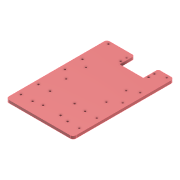
# Autodesk Inventor part: base plate
Saved by Autodesk Inventor 2022 (Build 260153000, 153)
## iProperties
Created: 2024-03-20
Part Number: base plate
Material: Generic
Document SubType Name: Modeling
Designer: david
Density: 1 g/cm^3
Appearance: Smooth - Red
Author: david
Autodesk Inventor part; units mm, degrees
ref_plane "YZ Plane" through (0, 0, 0) normal (1, 0, 0) x (0, 1, 0)
ref_plane "XZ Plane" through (0, 0, 0) normal (0, 1, 0) x (-1, 0, 0)
ref_plane "XY Plane" through (0, 0, 0) normal (0, 0, 1) x (1, 0, 0)
sketch "Sketch1" plane through (0, 0, 0) normal (0, 1, 0) x (-1, 0, 0)
  line L0 (57.5, -173) -> (57.5, -173) construction
  line L1 (-57.5, -173) -> (-57.5, 0) construction
  line L2 (-57.5, 0) -> (57.5, 0)
  line L3 (57.5, 0) -> (57.5, -173) construction
  line L4 (80.5, 0) -> (-80.5, 0) construction
  line L5 (0, -207.6) -> (0, 34.6) construction
  line L6 (57.5, -173) -> (-57.5, -173)
  line L7 (-57.5, -173) -> (-57.5, -173) construction
  line L8 (-57.5, 0) -> (57.5, 0)
  line L9 (57.5, 0) -> (57.5, -40)
  line L10 (-57.5, -40) -> (-57.5, 0)
  line L11 (57.5, -40) -> (57.5, -173)
  line L12 (-57.5, -173) -> (-57.5, -40)
  point P0 (0, 0)
  dimension "width" = 115
  dimension "Length" = 173
  dimension "d2" = 115
  constraints: 22 end point, 5 parallel, 4 horizontal, 4 perpendicular, 1 collinear, 1 point on line, 1 symmetric about line, 1 vertical alignment, 1 other
  measures "width" distance of L1.end L2.end
  measures "Length" distance of L1.start L1.end
  measures "d2" distance of L6.end L0.end
extrude "Base" add sketch "Sketch1" against normal blind 5
sketch "Sketch2" plane through (0, 0, 0) normal (0, 1, 0) x (1, 0, 0)
  line L0 (30, 48) -> (50, 48) construction
  line L1 (50, 48) -> (50, 18) construction
  line L2 (50, 18) -> (30, 18) construction
  line L3 (30, 18) -> (30, 48) construction
  line L4 (0, 207.6) -> (0, -34.6) construction
  line L5 (-30, 48) -> (-50, 48) construction
  line L6 (-50, 48) -> (-50, 18) construction
  line L7 (-50, 18) -> (-30, 18) construction
  line L8 (-30, 18) -> (-30, 48) construction
  line L9 (-57.5, 0) -> (57.5, 0) projected
  line L10 (-35, 53) -> (-25, 53) construction
  line L11 (-25, 53) -> (-25, 13) construction
  line L12 (-25, 13) -> (-35, 13) construction
  line L13 (-35, 13) -> (-35, 53) construction
  line L14 (-30, 43) -> (-30, 23) construction
  line L15 (30, 18) -> (30, 48) construction
  line L16 (35, 53) -> (25, 53) construction
  line L17 (25, 53) -> (25, 13) construction
  line L18 (25, 13) -> (35, 13) construction
  line L19 (35, 13) -> (35, 53) construction
  line L20 (30, 43) -> (30, 23) construction
  point P0 (0, 0)
  point P1 (-30, 53)
  point P2 (-30, 33)
  point P3 (-25, 33)
  point P4 (-30, 33)
  point P5 (30, 53)
  point P6 (30, 33)
  point P7 (25, 33)
  point P8 (30, 33)
  dimension "d5" = 20
  dimension "d6" = 30
  dimension "d8" = 18
  dimension "d16" = 10
  dimension "d18" = 20
  dimension "d19" = 10
  dimension "d20" = 50
  constraints: 38 end point, 18 symmetric about line, 8 coincident, 4 midpoint, 4 parallel, 4 point on line, 2 horizontal, 2 perpendicular, 1 horizontal alignment, 1 vertical alignment
  measures "d5" distance of L1.end L2.end
  measures "d6" distance of L0.end L1.end
  measures "d8" distance between parallel lines of L9 L2
  measures "d16" distance of L10.start L10.end
  measures "d18" distance of L14.end L14.start
  measures "d19" vertical distance of L10.end L14.start
  measures "d20" distance between parallel lines of L17 L11
hole "Bearing Holder Mounting Holes" at (30, 0, -48) at (50, 0, -48) at (50, 0, -18) at (-50, 0, -18) at (-30, 0, -48) at (-50, 0, -48) at (-30, 0, -18) at (30, 0, -18) direction (0, -1, 0) diameter 3.4 end through all
fillet "Fillet1" radius 5 4 edges at (57.5, -2.5, 0) (57.5, -2.5, -173) (-57.5, -2.5, -173) (-57.5, -2.5, 0)
sketch "Sketch5" plane through (0, 0, 0) normal (0, 1, 0) x (1, 0, 0)
  line L0 (-34.5, 80) -> (34.5, 80) construction
  line L1 (34.5, 80) -> (34.5, 114) construction
  line L2 (34.5, 114) -> (-34.5, 114) construction
  line L3 (-34.5, 114) -> (-34.5, 80) construction
  line L4 (-57.5, 0) -> (52.5, 0) projected
  point P0 (0, 0)
  point P1 (-52.2987, 0)
  point P2 (0, 80)
  dimension "d41" = 34
  dimension "d42" = 69
  dimension "d43" = 80
  constraints: 8 end point, 2 parallel, 1 horizontal, 1 midpoint, 1 perpendicular, 1 vertical alignment
  measures "d41" distance of L2.end L0.start
  measures "d42" distance of L1.end L2.end
  measures "d43" distance between parallel lines of L4 L0
hole "12v Motor Mount Mounting Holes" at (-34.5, 0, -114) at (-34.5, 0, -80) at (34.5, 0, -80) at (34.5, 0, -114) direction (0, -1, 0) diameter 3.2 end through all
sketch "Sketch8" plane through (0, 0, 0) normal (0, 1, 0) x (1, 0, 0)
  line L0 (-10, 148) -> (30, 148)
  line L1 (30, 148) -> (30, 168)
  line L2 (30, 168) -> (-10, 168)
  line L3 (-10, 168) -> (-10, 148)
  line L4 (52.5, 173) -> (-52.5, 173) projected
  line L5 (-57.5, 0) -> (52.5, 0) projected
  line L6 (-52.5, 173) -> (52.5, 173) projected
  line L7 (-10, 168) -> (30, 168)
  line L8 (30, 168) -> (30, 173)
  line L9 (30, 173) -> (-10, 173)
  line L10 (-10, 173) -> (-10, 168)
  point P0 (0, 0)
  point P1 (0, 173)
  point P2 (30, 170.5)
  dimension "d64" = 20
  dimension "d65" = 40
  dimension "d67" = 10
  dimension "d147" = 5
  constraints: 16 end point, 4 parallel, 2 horizontal, 2 midpoint, 2 perpendicular, 1 point on line, 1 vertical alignment
  measures "d64" distance of L2.end L0.start
  measures "d65" distance of L1.end L2.end
  measures "d67" distance from line of point (0, 173) L3
  measures "d147" distance between parallel lines of L4 L2
extrude "Servo Cutout 2" cut sketch "Sketch8" against normal through all
sketch "Sketch9" plane through (0, 0, 0) normal (0, 1, 0) x (1, 0, 0)
  line L0 (-13.925, 153) -> (33.925, 153) construction
  line L1 (33.925, 153) -> (33.925, 163) construction
  line L2 (33.925, 163) -> (-13.925, 163) construction
  line L3 (-13.925, 163) -> (-13.925, 153) construction
  line L4 (30, 168) -> (30, 148) construction
  line L5 (-10, 148) -> (-10, 168) construction
  point P0 (0, 0)
  point P1 (-10, 158)
  point P2 (-13.925, 158)
  point P3 (-10, 158)
  dimension "d70" = 3.925
  dimension "d71" = 5
  dimension "d72" = 3.925
  constraints: 8 end point, 3 midpoint, 2 parallel, 1 horizontal, 1 horizontal alignment, 1 perpendicular
  measures "d70" distance between parallel lines of L1 L4
  measures "d71" vertical distance of L2.end point (-10, 158)
  measures "d72" distance between parallel lines of L5 L3
hole "Servo Mounting Holes 2" at (-13.925, 0, -153) at (-13.925, 0, -163) at (33.925, 0, -153) at (33.925, 0, -163) direction (0, -1, 0) diameter 3.4 end through all
sketch "Sketch10" plane through (0, 0, 0) normal (0, 1, 0) x (1, 0, 0)
  circle A0 centre (34.5, 80) radius 1.6 construction
  circle A1 centre (-34.5, 114) radius 1.6 construction
  circle A2 centre (-34.5, 80) radius 1.6 construction
  circle A3 centre (34.5, 114) radius 1.6 construction
  arc A4 (52.5, 0) -> (57.5, 5) centre (52.5, 5) ccw construction
  line L0 (52.5, 0) -> (-52.5, 0) construction
  line L1 (-57.5, 5) -> (-57.5, 168) construction
  line L2 (-52.5, 173) -> (-10, 173) construction
  line L3 (57.5, 168) -> (57.5, 5) construction
  circle A5 centre (-30, 18) radius 1.7 construction
  circle A6 centre (-30, 48) radius 1.7 construction
  circle A7 centre (50, 18) radius 1.7 construction
  circle A8 centre (30, 48) radius 1.7 construction
  circle A9 centre (50, 48) radius 1.7 construction
  circle A10 centre (-50, 18) radius 1.7 construction
  circle A11 centre (-50, 48) radius 1.7 construction
  circle A12 centre (30, 18) radius 1.7 construction
  line L4 (0, 209.0497) -> (0, -36.0497) construction
  arc A13 (-52.5, 173) -> (-57.5, 168) centre (-52.5, 168) ccw projected
  arc A14 (57.5, 168) -> (52.5, 173) centre (52.5, 168) ccw projected
  arc A15 (-57.5, 5) -> (-52.5, 0) centre (-52.5, 5) ccw projected
  circle A16 centre (33.925, 153) radius 1.7 projected
  circle A17 centre (-13.925, 153) radius 1.7 projected
  circle A18 centre (-13.925, 163) radius 1.7 projected
  circle A19 centre (33.925, 163) radius 1.7 projected
  line L5 (-10, 148) -> (30, 148) projected
  line L6 (-10, 173) -> (-10, 148) projected
  line L7 (30, 148) -> (30, 173) projected
  line L8 (30, 173) -> (52.5, 173) projected
  point P0 (-50, 168)
  point P1 (50, 168)
  dimension "d93" = 5
  dimension "d94" = 50
  dimension "d111" = 50
  constraints: 1 symmetric about line
  measures "d93" distance from line of L2 point (-50, 168)
  measures "d94" distance from line of L4 point (-50, 168)
  measures "d111" distance from line of A10.centre L4
hole "Extra Holes For Top Plate" at (-50, 0, -168) at (50, 0, -168) direction (0, -1, 0) diameter 3.4 depth 6
sketch "Sketch11" plane through (0, 0, 0) normal (0, 1, 0) x (1, 0, 0)
  line L0 (49.5, 123) -> (49.5, 93) construction
  line L1 (52.5, 173) -> (-52.5, 173) construction
  line L2 (0, 207.6) -> (0, -34.6) projected
  line L3 (-49.5, 123) -> (-49.5, 93) construction
  line L4 (15, 21) -> (-15, 21)
  line L5 (57.5, 5) -> (57.5, 168) projected
  line L6 (-52.5, 0) -> (52.5, 0) projected
  point P0 (0, 0)
  point P1 (0, 21)
  point P2 (0, 173)
  dimension "d95" = 50
  dimension "d96" = 30
  dimension "d108" = 30
  dimension "d110" = 8
  dimension "d146" = 21
  constraints: 6 coincident, 6 end point, 4 symmetric about line, 2 midpoint, 1 horizontal, 1 parallel, 1 vertical alignment
  measures "d95" distance from line of L1 L0.start
  measures "d96" distance of L0.start L0.end
  measures "d108" distance of L4.start L4.end
  measures "d110" distance between parallel lines of L5 L0
  measures "d146" distance between parallel lines of L6 L4
hole "Ultrasonic Sensor Mounting Holes" at (49.5, 0, -123) at (49.5, 0, -93) at (-49.5, 0, -93) at (-49.5, 0, -123) at (-15, 0, -21) at (15, 0, -21) direction (0, -1, 0) diameter 3.4 depth 6
thicken "Clearance for Servo" operation add thickness 0.5 both sides no extend neighbours yes toward (0, 0, 1) faces at (3.3333, -1.6667, -148) (-10, -1.6667, -164.6667) (30, -1.6667, -156.3333)
sketch "Sketch13" plane through (0, 0, 0) normal (0, -1, 0) x (1, 0, 0)
  line L0 (-15, -60.5) -> (15, -60.5)
  line L1 (52.5, 0) -> (-52.5, 0) projected
  point P0 (0, 0)
  point P1 (0, -60.5)
  point P2 (-57.5, 0)
  dimension "d124" = 60.5
  constraints: 2 coincident, 2 end point, 1 horizontal, 1 horizontal alignment, 1 midpoint, 1 vertical alignment
  measures "d124" distance between parallel lines of L1 L0
hole "Driver Gear Stopper Mounting Holes" [suppressed]
fillet "Fillet2" radius 3 2 edges at (30.5, -2.5, -173) (-10.5, -2.5, -173)
sketch "Sketch16" plane through (0, -5, 0) normal (0, -1, 0) x (1, 0, 0)
  line L0 (6, -55) -> (21, -55)
  line L1 (21, -55) -> (21, -68)
  line L2 (21, -68) -> (6, -68)
  line L3 (6, -68) -> (6, -55)
  line L4 (6, -55) -> (21, -68) construction
  line L5 (21, -55) -> (6, -68) construction
  line L6 (6, -44.9548) -> (6, -85.5548)
  line L7 (9.5, -50.5) -> (9.5, -72.5) construction
  line L8 (6, -50.5) -> (6, -55) construction
  line L9 (13, -72.5) -> (13, -55)
  arc A0 (13, -50.5) -> (6, -50.5) centre (9.5, -50.5) ccw construction
  arc A1 (6, -72.5) -> (13, -72.5) centre (9.5, -72.5) ccw
  line L10 (6, -55) -> (6, -72.5)
  line L11 (13, -55) -> (13, -50.5) construction
  circle A2 centre (34.5, -80) radius 1.6 projected
  line L12 (21, -61.5) -> (6, -61.5)
  point P0 (0, 0)
  point P1 (11.8839, -63.9814)
  point P2 (13.5, -61.5)
  point P3 (6, -44.9548)
  point P4 (6, -85.5548)
  point P5 (13.5, -61.5)
  point P6 (9.5, -61.5)
  dimension "d149" = 13
  dimension "d150" = 15
  dimension "d151" = 7
  dimension "d152" = 8
  dimension "d153" = 8
  dimension "d163" = 12
  dimension "d164" = 6
  constraints: 26 end point, 8 tangent, 7 parallel, 5 midpoint, 4 point on circle, 2 centre point, 2 coincident, 2 collinear, 2 perpendicular, 1 point on line, 1 vertical, 4 other
  measures "d149" distance of L5.end L4.start
  measures "d150" distance of L4.end L5.end
  measures "d151" diameter of A1
  measures "d163" distance from line of L2 A2.centre
hole "Optical sensor holes" at (9.5, -5, -50.5) direction (0, 1, 0) diameter 3.4 end through all
sketch "Sketch15" plane through (0, 0, 0) normal (0, 1, 0) x (1, 0, 0)
  circle A0 centre (-30, 48) radius 1.7 projected
  circle A1 centre (-30, 18) radius 1.7 projected
  circle A2 centre (30, 48) radius 1.7 projected
  circle A3 centre (30, 18) radius 1.7 projected
  point P0 (0, 0)
  constraints: 4 coincident
equation "\"d2\" = width"
equation "\"d9\" = HoleDia"
equation "\"d72\" = d70"
equation "\"d73\" = HoleDia"
equation "\"d94\" = d111"
equation "\"d84\" = HoleDia"
equation "\"d98\" = HoleDia"
equation "\"d100\" = CBORE"
equation "\"d125\" = HoleDia"
equation "\"d127\" = CBORE"
equation "\"d153\" = d152"
equation "\"HoleDia\" = 3.4"
equation "\"CBORE\" = 7"
body "Solid1"
